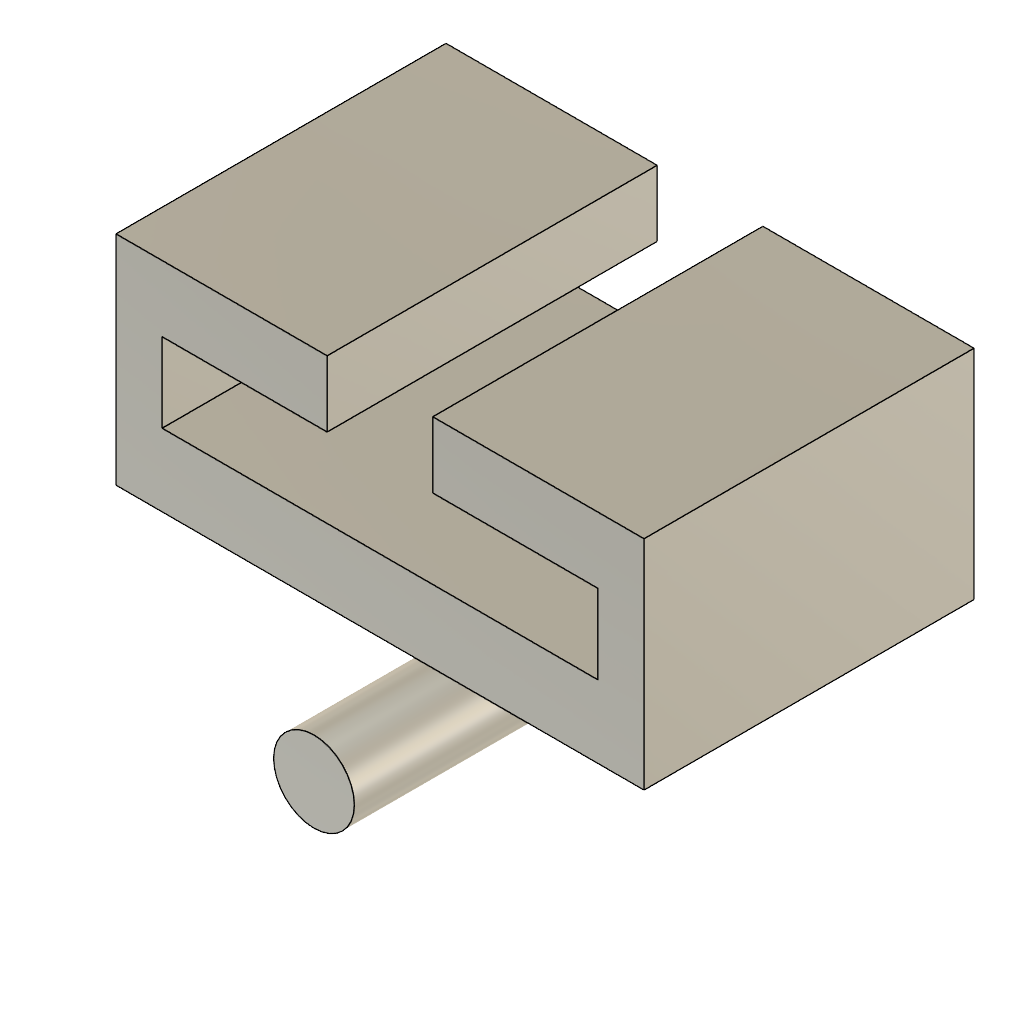
Bracket_Mount (Autodesk Fusion 360 design; units mm, degrees)
part number: 2026-09-23-19-24-28-696
Autodesk Fusion 360 part; units mm, degrees
note: some values were not read from the file. Set by a fixed rule: which sketch regions a step uses.
sketch "Sketch1" plane through (0, 0, 0) normal (0, 1, 0) x (1, 0, 0)
  circle A0 centre (0, 0) radius 7.7724
  dimension "d1" = 15.5448
  constraint coincident A0.centre origin
  measures "d1" diameter of A0
extrude "Extrude1" add sketch "Sketch1" along normal blind 76.2
sketch "Sketch2" plane through (0, 76.2, 0) normal (0, 1, 0) x (-1, 0, 0)
  circle A0 centre (0, 0) radius 7.7724
  line L0 (-7.7723, 0.0299) -> (7.7725, 0.0299)
  line L1 (7.7725, 0.0299) -> (7.7725, 17.6304)
  line L2 (7.7725, 17.6304) -> (-7.7723, 17.6304)
  line L3 (-7.7723, 17.6304) -> (-7.7723, 0.0299)
  dimension "d4" = 15.5448
  constraint horizontal L0
  constraint vertical L1
  constraint horizontal L2
  constraint vertical L3
  constraint coincident A0 L0.start
  measures "d4" distance of L0.start L0.end
extrude "Extrude2" add sketch "Sketch2" against normal blind 6.35 contours A0 L1 L2 L3
sketch "Sketch3" plane through (0, 0, 17.6304) normal (0, 0, 1) x (-1, 0, 0)
  line L0 (-7.7723, -76.2) -> (7.7725, -76.2)
  line L1 (7.7725, -76.2) -> (7.7725, -69.85)
  line L2 (7.7725, -69.85) -> (-7.7723, -69.85)
  line L3 (-7.7723, -69.85) -> (-7.7723, -76.2)
  line L4 (-50.8, -76.2) -> (50.8, -76.2)
  line L5 (50.8, -76.2) -> (50.8, -12.7)
  line L6 (50.8, -12.7) -> (-50.8, -12.7)
  line L7 (-50.8, -12.7) -> (-50.8, -76.2)
  dimension "d7" = 101.6
  dimension "d8" = 63.5
  constraint horizontal L4
  constraint vertical L5
  constraint horizontal L6
  constraint vertical L7
  measures "d7" distance of L4.start L4.end
  measures "d8" distance of L4.start L6.end
extrude "Extrude3" add sketch "Sketch3" along normal blind 21.5646
sketch "Sketch4" plane through (0, 0, 39.195) normal (0, 0, 1) x (-1, 0, 0)
  line L0 (-50.8, -12.7) -> (-50.8, -76.2)
  line L1 (-50.8, -76.2) -> (50.8, -76.2)
  line L2 (50.8, -76.2) -> (50.8, -12.7)
  line L3 (50.8, -12.7) -> (-50.8, -12.7)
  line L4 (50.8, -12.7) -> (41.91, -12.7)
  line L5 (41.91, -12.7) -> (41.91, -76.2)
  line L6 (41.91, -76.2) -> (50.8, -76.2)
  line L7 (50.8, -76.2) -> (50.8, -12.7)
  line L8 (-50.8, -76.2) -> (-41.91, -76.2)
  line L9 (-41.91, -76.2) -> (-41.91, -12.7)
  line L10 (-41.91, -12.7) -> (-50.8, -12.7)
  line L11 (-50.8, -12.7) -> (-50.8, -76.2)
  dimension "d11" = 8.89
  dimension "d12" = 63.5
  dimension "d13" = 8.89
  constraint horizontal L4
  constraint vertical L5
  constraint horizontal L6
  constraint vertical L7
  constraint coincident L2.end L3.start
  constraint horizontal L8
  constraint vertical L9
  constraint horizontal L10
  constraint vertical L11
  constraint coincident L0.end L1.start
  measures "d11" distance of L2.end L4.end
  measures "d12" distance of L2.end L1.end
  measures "d13" distance of L0.end L8.end
extrude "Extrude4" add sketch "Sketch4" along normal blind 20.32 contours L0 L1 L3 L8 L9 L10 L11 | L1 L2 L3 L4 L5 L6 L7
sketch "Sketch5" plane through (-41.91, 0, 0) normal (1, 0, 0) x (0, 1, 0)
  line L0 (12.7, 39.195) -> (76.2, 39.195)
  line L1 (76.2, 39.195) -> (76.2, 59.515)
  line L2 (76.2, 59.515) -> (12.7, 59.515)
  line L3 (12.7, 59.515) -> (12.7, 39.195)
  line L4 (12.7, 59.515) -> (76.2, 59.515)
  line L5 (76.2, 59.515) -> (76.2, 54.435)
  line L6 (76.2, 54.435) -> (12.7, 54.435)
  line L7 (12.7, 54.435) -> (12.7, 59.515)
  dimension "d16" = 63.5
  dimension "d17" = 5.08
  constraint horizontal L4
  constraint vertical L5
  constraint horizontal L6
  constraint vertical L7
  constraint coincident L2.end L3.start
  measures "d16" distance of L2.end L1.end
  measures "d17" distance of L2.end L6.end
sketch "Sketch6" plane through (41.91, 0, 0) normal (-1, 0, 0) x (0, -1, 0)
  line L0 (-76.2, 39.195) -> (-12.7, 39.195)
  line L1 (-12.7, 39.195) -> (-12.7, 59.515)
  line L2 (-12.7, 59.515) -> (-76.2, 59.515)
  line L3 (-76.2, 59.515) -> (-76.2, 39.195)
  line L4 (-76.2, 59.515) -> (-12.7, 59.515)
  line L5 (-12.7, 59.515) -> (-12.7, 54.435)
  line L6 (-12.7, 54.435) -> (-76.2, 54.435)
  line L7 (-76.2, 54.435) -> (-76.2, 59.515)
  dimension "d18" = 63.5
  dimension "d19" = 5.08
  constraint horizontal L4
  constraint vertical L5
  constraint horizontal L6
  constraint vertical L7
  constraint coincident L2.end L3.start
  measures "d18" distance of L2.end L1.end
  measures "d19" distance of L2.end L6.end
extrude "Extrude5" add sketch "Sketch5" along normal blind 31.75 contours L1 L2 L3 L4 L5 L6 L7
sketch "Sketch7" plane through (41.91, 0, 0) normal (-1, 0, 0) x (0, -1, 0)
extrude "Extrude6" add sketch "Sketch6" along normal blind 31.75 contours L1 L2 L3 L4 L5 L6 L7
extrude "Extrude7" cut 1 faces at (2.5908, 33.8667, 39.195) along direction (0, 0, -1) blind 7.62
extrude "Extrude8" add 2 faces at (-31.3267, 55.0333, 54.435) (31.3267, 33.8667, 54.435) along direction (0, 0, -1) blind 7.62
